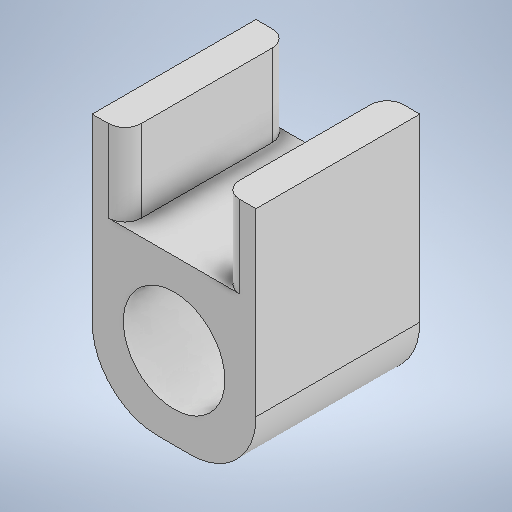
# Autodesk Inventor part: gomu_guide2.8
Saved by Autodesk Inventor 2025 (Build 290162000, 162)
## iProperties
Created: 2024-07-18
Part Number: gomu_guide2.8
Material: 一般
Document SubType Name: Modeling
Designer: Akio
Density: 1 g/cm^3
Appearance: 既定
Author: Akio
Autodesk Inventor part; units mm, degrees
ref_plane "YZ Plane" through (0, 0, 0) normal (1, 0, 0) x (0, 1, 0)
ref_plane "XZ Plane" through (0, 0, 0) normal (0, 1, 0) x (-1, 0, 0)
ref_plane "XY Plane" through (0, 0, 0) normal (0, 0, 1) x (1, 0, 0)
sketch "スケッチ1" plane through (0, 0, 0) normal (0, 1, 0) x (-1, 0, 0)
  line L0 (0, 0) -> (-5, 0)
  line L1 (-5, 0) -> (-5, -5)
  line L2 (-5, -5) -> (0, -5)
  line L3 (0, -5) -> (0, 0)
  dimension "d0" = 5
  dimension "d1" = 5
  constraints: 8 end point, 2 parallel, 1 horizontal, 1 perpendicular
  measures "d0" distance of L2.end L1.end
  measures "d1" distance of L1.end L0.end
extrude "押し出し1" add sketch "スケッチ1" along normal blind 7.5
sketch "スケッチ2" plane through (0, 0, 0) normal (0, 0, 1) x (1, 0, 0)
  line L0 (0, 0) -> (5, 0) projected
  line L1 (0, 0) -> (0, 7.5) projected
  point P0 (2.5, 2.5)
  dimension "d11" = 2.5
  dimension "d12" = 2.5
  measures "d11" distance from line of L0 point (2.5, 2.5)
  measures "d12" distance from line of L1 point (2.5, 2.5)
hole "穴1" at (2.5, 2.5, 0) direction (0, 0, -1) diameter 3.1 end through all
sketch "スケッチ3" plane through (0, 0, 0) normal (0, 0, 1) x (1, 0, 0)
  line L0 (1, 7.5) -> (4, 7.5)
  line L1 (4, 7.5) -> (4, 5)
  line L2 (4, 5) -> (1, 5)
  line L3 (1, 5) -> (1, 7.5)
  line L4 (1, 7.5) -> (4, 5) construction
  line L5 (4, 7.5) -> (1, 5) construction
  line L6 (0, 0) -> (0, 7.5) projected
  line L7 (0, 7.5) -> (5, 7.5) projected
  point P0 (2.5, 6.25)
  dimension "d13" = 3
  dimension "d14" = 2.5
  dimension "d15" = 2.5
  dimension "d16" = 0
  constraints: 12 end point, 2 midpoint, 2 parallel, 1 horizontal, 1 perpendicular
  measures "d13" distance of L1.end L2.end
  measures "d14" distance of L0.end L1.end
  measures "d15" distance from line of L6 point (2.5, 6.25)
  measures "d16" distance between parallel lines of L0 L7
extrude "押し出し2" cut sketch "スケッチ3" against normal through all
fillet "フィレット1" radius 2 2 edges at (5, 0, -2.5) (0, 0, -2.5)
fillet "フィレット2" radius 0.5 4 edges at (1, 6.25, 0) (4, 6.25, 0) (1, 6.25, -5) (4, 6.25, -5)
equation "\"d12\" = 0.5 * d0"
equation "\"d15\" = 0.5 * d0"
